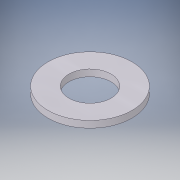
# Autodesk Inventor part: .125 washer
Saved by Autodesk Inventor 2017 (Build 210142000, 142)
## iProperties
Created: 2017-04-26
Part Number: .125 washer
Material: Aluminum 6061, Welded
Document SubType Name: Modeling
Designer: Delta
Density: 2.7 g/cm^3
Appearance: Weld - Aluminum
Mass: 0.00407227 g
Surface Area: 0.156763 cm^2
Volume: 0.00150825 cm^3
Author: Delta
Autodesk Inventor part; units mm, degrees
ref_plane "YZ Plane" through (0, 0, 0) normal (1, 0, 0) x (0, 1, 0)
ref_plane "XZ Plane" through (0, 0, 0) normal (0, 1, 0) x (-1, 0, 0)
ref_plane "XY Plane" through (0, 0, 0) normal (0, 0, 1) x (1, 0, 0)
sketch "Sketch1" plane through (0, 0, 0) normal (0, 1, 0) x (-1, 0, 0)
  circle A0 centre (0, 0) radius 1.5875
  dimension "d0" = 3.175
  constraints: 1 centre point, 1 coincident
  measures "d0" diameter of A0
extrude "Extrusion1" add sketch "Sketch1" along normal blind 0.254
hole "Hole1" at (0, 0, 0) direction (0, 1, 0) diameter 1.5875 depth 1.5875 tip angle 118
body "Solid1"
